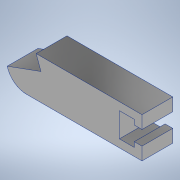
# Autodesk Inventor part: Finray_test_8_Kerbe_10deg
Saved by Autodesk Inventor 2022 (Build 260153000, 153)
## iProperties
Created: 2022-02-28
Part Number: Finray_test_8_Kerbe_10deg
Material: Generic
Document SubType Name: Modeling
Designer: richa
Density: 1 g/cm^3
Appearance: Aluminum - Flat
Author: richa
Autodesk Inventor part; units mm, degrees
ref_plane "YZ Plane" through (0, 0, 0) normal (1, 0, 0) x (0, 1, 0)
ref_plane "XZ Plane" through (0, 0, 0) normal (0, 1, 0) x (-1, 0, 0)
ref_plane "XY Plane" through (0, 0, 0) normal (0, 0, 1) x (1, 0, 0)
sketch "Sketch5" plane through (0, 0, 0) normal (0, 0, 1) x (1, 0, 0)
  line L0 (52.8, -15.6) -> (52.8, -10.6)
  line L1 (52.8, -10.6) -> (49.8, -10.6)
  line L2 (49.8, -10.6) -> (49.8, -12.55)
  line L3 (44, -12.55) -> (44, -3.05)
  line L4 (49.8, -3.05) -> (49.8, -5)
  line L5 (49.8, -5) -> (52.8, -5)
  line L6 (52.8, -5) -> (52.8, 0)
  line L7 (52.8, 0) -> (7.8, 0)
  line L8 (44, -3.05) -> (49.8, -3.05)
  line L9 (44, -12.55) -> (49.8, -12.55)
  line L10 (52.8, -15.6) -> (7.8, -15.6)
  arc A0 (7.8, 0) -> (7.8, -15.6) centre (7.8, -7.8) ccw
  point P0 (0, 0)
  dimension "d41" = 5.8
  dimension "d48" = 44
  dimension "d63" = 45
  dimension "d67" = 15.6
  dimension "d71" = 0
  dimension "d72" = 36.2
  dimension "d85" = 5.6
  dimension "d86" = 9.5
  dimension "d87" = 3
  constraints: 22 end point, 7 perpendicular, 4 collinear, 2 parallel, 2 point on circle, 2 tangent, 1 centre point, 1 horizontal, 1 vertical
  measures "d41" distance between parallel lines of L2 L3
  measures "d48" distance from line of L3 point (0, 0)
  measures "d63" distance of L0.start L10.end
  measures "d67" diameter of A0
  measures "d71" distance from line of point (0, 0) L7
  measures "d72" distance from line of L3 A0.centre
  measures "d85" distance between parallel lines of L1 L5
  measures "d86" distance of L3.start L3.end
  measures "d87" distance of L4.end L5.end
extrude "Extrusion2" add sketch "Sketch5" along normal blind 12
sketch "Sketch8" plane through (0, 0, 0) normal (0, 0, -1) x (-1, 0, 0)
  arc A0 (-7.8, -15.6) -> (-7.8, 0) centre (-7.8, -7.8) ccw projected
  line L0 (-11.5745, 0) -> (-13.6398, -5.6745)
  line L1 (-7.8, 0) -> (-1.143, 0) construction
  arc A1 (-7.8, -15.6) -> (-7.8, 0) centre (-7.8, -7.8) ccw projected
  line L2 (-7.8, -7.8) -> (4.6142, -7.8) construction
  line L3 (1.0278, -11.0131) -> (-7.8, -7.8) construction
  line L4 (-7.8, -7.8) -> (-17.6382, -4.2192) construction
  line L5 (-52.8, 0) -> (-7.8, 0) projected
  arc A2 (-0.2769, -9.8933) -> (-7.8, 0) centre (-7.7907, -7.8) ccw
  line L6 (-0.2769, -9.8933) -> (-13.4326, -5.105)
  line L7 (-52.8, 0) -> (-7.8, 0) projected
  arc A3 (-0.2769, -9.8933) -> (-7.8, 0) centre (-7.7907, -7.8) ccw
  line L8 (-7.8, 0) -> (-11.5745, 0)
  point P0 (0, 0)
  point P1 (-0.2853, -9.8902)
  dimension "d80" = 110
  dimension "d81" = 20
  dimension "d84" = 20
  dimension "d88" = 14
  constraints: 14 end point, 4 point on circle, 4 point on line, 2 centre point, 2 horizontal, 1 equal radius, 1 perpendicular
  measures "d80" angle of L0 L1
  measures "d81" angle of L2 L3
  measures "d84" angle of L2 L6
  measures "d88" distance of L6.start L6.end
extrude "Extrusion5" cut sketch "Sketch8" against normal through all
equation "\"l1\" = 8"
body "Solid2"
